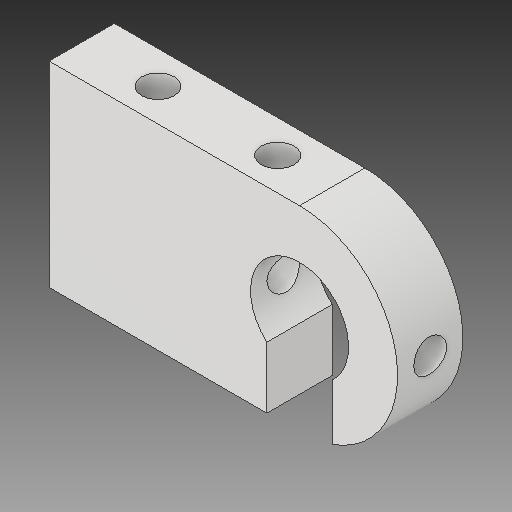
# Autodesk Inventor part: Hand - Digit 2-3
Saved by Autodesk Inventor 2017 (Build 210142000, 142)
## iProperties
Created: 2016-09-27
Part Number: Hand - Digit 2-3
Material: ABS Plastic
Document SubType Name: Modeling
Designer: cmcdona
Density: 1.06 g/cm^3
Appearance: Smooth - White
Author: cmcdona
Autodesk Inventor part; units mm, degrees
ref_plane "YZ Plane" through (0, 0, 0) normal (1, 0, 0) x (0, 1, 0)
ref_plane "XZ Plane" through (0, 0, 0) normal (0, 1, 0) x (-1, 0, 0)
sketch "Sketch1" plane through (0, 0, 0) normal (0, 0, 1) x (1, 0, 0)
  line L0 (0, 0) -> (23, 0)
  arc A0 (23, 0) -> (23, 18) centre (23, 9) ccw
  line L1 (23, 18) -> (0, 18)
  line L2 (0, 18) -> (0, 0)
  circle A1 centre (23, 9) radius 4.5
  dimension "d0" = 23
  dimension "d1" = 18
  dimension "d2" = 9
  dimension "d3" = 9
  constraints: 6 end point, 2 centre point, 2 horizontal, 2 point on circle, 1 coincident, 1 perpendicular
  measures "d0" distance of L0.start L0.end
  measures "d1" distance of L0.end L1.start
  measures "d2" radius of A0
  measures "d3" diameter of A1
extrude "Extrusion1" add sketch "Sketch1" against normal blind 6
sketch "Sketch2" plane through (0, 18, 0) normal (0, 1, 0) x (1, 0, 0)
  circle A0 centre (18, 3) radius 1.5
  circle A1 centre (7, 3) radius 1.5
  point P0 (0, 0)
  dimension "d6" = 3
  dimension "d7" = 3
  constraints: 2 centre point
  measures "d6" diameter of A0
  measures "d7" diameter of A1
extrude "Extrusion2" cut sketch "Sketch2" against normal blind 5
sketch "Sketch3" plane through (0, 0, 0) normal (0, 0, 1) x (1, 0, 0)
  line L0 (20, 0) -> (26, 0)
  line L1 (26, 0) -> (26, 6)
  line L2 (26, 6) -> (20, 6)
  line L3 (20, 6) -> (20, 0)
  point P0 (0, 0)
  dimension "d10" = 6
  dimension "d11" = 6
  constraints: 8 end point, 2 parallel, 1 horizontal, 1 perpendicular
  measures "d10" distance of L2.end L1.end
  measures "d11" distance of L1.end L0.end
extrude "Extrusion3" cut sketch "Sketch3" against normal through all
ref_plane "Work Plane1" through (32, 0, 0) normal (-1, 0, 0) x (0, 0, 1)
sketch "Sketch4" plane through (32, 0, 0) normal (-1, 0, 0) x (0, 0, 1)
  circle A0 centre (-3, 9) radius 1.5
  point P0 (0, 0)
  dimension "d15" = 3
  constraints: 1 centre point
  measures "d15" diameter of A0
extrude "Extrusion4" cut sketch "Sketch4" along normal blind 18
body "Solid1"
